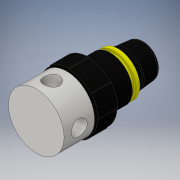
# Autodesk Inventor part: 101-3002-1
Saved by Autodesk Inventor 2016 SP2 (Build 200236200, 236)
## iProperties
Created: 2017-03-30
Part Number: 101-3002-1
Material: Aluminum
Document SubType Name: Modeling
Designer: smiku
Mass: 129.93 g
Surface Area: 139.496 cm^2
Volume: 48.1222 cm^3
Density: 2.7 g/cm^3
Appearance: Satin
Author: smiku
Autodesk Inventor part; units mm, degrees
ref_plane "YZ Plane" through (0, 0, 0) normal (1, 0, 0) x (0, 1, 0)
ref_plane "XY Plane" through (0, 0, 0) normal (0, 0, 1) x (1, 0, 0)
sketch "Sketch1" plane through (0, 0, 0) normal (0, 0, 1) x (1, 0, 0)
  circle A0 centre (0, 0) radius 17.9959
  dimension "d0" = 35.9918
  constraints: 1 centre point, 1 coincident
  measures "d0" diameter of A0
extrude "Extrusion1" add sketch "Sketch1" along normal blind 19.7358
sketch "Sketch2" plane through (0, 0, 0) normal (0, 0, -1) x (-1, 0, 0)
  circle A0 centre (0, 0) radius 12.7
  dimension "d3" = 25.4
  constraints: 1 centre point, 1 coincident
  measures "d3" diameter of A0
extrude "Extrusion2" add sketch "Sketch2" along normal blind 1.27
sketch "Sketch3" plane through (0, 0, -1.27) normal (0, 0, -1) x (-1, 0, 0)
  circle A0 centre (0, 0) radius 18.6055
  arc A1 (12.2451, 14.5931) -> (0, 19.05) centre (0, 0) ccw
  line L0 (0, 0) -> (12.2451, 14.5931) construction
  line L1 (0, 0) -> (0, 19.05) construction
  line L2 (0, 19.05) -> (0, 18.6055)
  line L3 (11.9594, 14.2526) -> (12.2451, 14.5931)
  arc A2 (11.9594, 14.2526) -> (0, 18.6055) centre (0, 0) ccw
  arc A3 (-14.5931, 12.2451) -> (-19.05, 0) centre (0, 0) ccw
  line L4 (-19.05, 0) -> (-18.6055, 0)
  arc A4 (-14.2526, 11.9594) -> (-18.6055, 0) centre (0, 0) ccw
  line L5 (-14.2526, 11.9594) -> (-14.5931, 12.2451)
  arc A5 (-12.2451, -14.5931) -> (0, -19.05) centre (0, 0) ccw
  line L6 (0, -19.05) -> (0, -18.6055)
  arc A6 (-11.9594, -14.2526) -> (0, -18.6055) centre (0, 0) ccw
  line L7 (-11.9594, -14.2526) -> (-12.2451, -14.5931)
  arc A7 (14.5931, -12.2451) -> (19.05, 0) centre (0, 0) ccw
  line L8 (19.05, 0) -> (18.6055, 0)
  arc A8 (14.2526, -11.9594) -> (18.6055, 0) centre (0, 0) ccw
  line L9 (14.2526, -11.9594) -> (14.5931, -12.2451)
  dimension "d6" = 37.211
  dimension "d7" = 19.05
  dimension "d8" = 40
  dimension "d11" = 360
  constraints: 20 end point, 18 point on circle, 9 centre point, 6 coincident, 2 point on line, 1 vertical, 41 other
  measures "d6" diameter of A0
  measures "d7" radius of A1
  measures "d8" angle of L0 L1
extrude "Extrusion3" add sketch "Sketch3" along normal blind 12.7 separate body
sketch "Sketch4" plane through (0, 0, -13.97) normal (0, 0, -1) x (-1, 0, 0)
  circle A0 centre (0, 0) radius 14.2875
  dimension "d15" = 28.575
  constraints: 1 centre point, 1 coincident
  measures "d15" diameter of A0
extrude "Extrusion4" add sketch "Sketch4" along normal blind 14.224 bodies 2
sketch "Sketch5" plane through (0, 0, -28.194) normal (0, 0, -1) x (-1, 0, 0)
  circle A0 centre (0, 0) radius 10.16
  dimension "d18" = 20.32
  constraints: 1 centre point, 1 coincident
  measures "d18" diameter of A0
extrude "Extrusion5" add sketch "Sketch5" along normal blind 10.16 bodies 2
sketch "Sketch6" plane through (0, 0, 0) normal (0, 1, 0) x (-1, 0, 0)
  line L0 (-10.16, -38.354) -> (10.16, -38.354) construction
  line L1 (0, -38.354) -> (11.7475, -38.354)
  line L2 (0, -38.354) -> (0, -49.784)
  line L3 (0, -49.784) -> (8.89, -49.784)
  arc A0 (8.89, -49.784) -> (10.795, -48.0569) centre (8.89, -47.8698) ccw
  line L4 (10.795, -48.0569) -> (11.7475, -38.354)
  point P0 (0, 0)
  dimension "d21" = 11.7475
  dimension "d22" = 11.43
  dimension "d23" = 8.89
  dimension "d24" = 10.795
  constraints: 8 end point, 2 horizontal, 2 point on circle, 2 tangent, 1 centre point, 1 midpoint, 1 vertical
  measures "d21" distance of L1.start L1.end
  measures "d22" distance of L1.start L2.end
  measures "d23" distance of L2.end L3.end
  measures "d24" distance from line of L2 L4.start
revolve "Revolution1" add sketch "Sketch6" angle 360 about axis through (0, 0, -38.354) along (0, 0, -1) bodies 2
sketch "Sketch7" plane through (0, 0, -28.194) normal (0, 0, -1) x (-1, 0, 0)
  circle A0 centre (0, 0) radius 10.16 projected
  circle A1 centre (0, 0) radius 12.7
  dimension "d26" = 25.4
  constraints: 1 centre point, 1 coincident
  measures "d26" diameter of A1
extrude "Extrusion6" add sketch "Sketch7" along normal blind 2.54 separate body
sketch "Sketch8" plane through (0, 0, -30.734) normal (0, 0, -1) x (-1, 0, 0)
  circle A0 centre (0, 0) radius 10.16 projected
  circle A1 centre (0, 0) radius 13.97
  dimension "d29" = 27.94
  constraints: 1 centre point, 1 coincident
  measures "d29" diameter of A1
extrude "Extrusion7" add sketch "Sketch8" along normal blind 2.54 bodies 3
ref_plane "Work Plane1" through (0, 17.9959, 0) normal (0, 1, 0) x (-1, 0, 0)
sketch "Sketch9" plane through (0, 17.9959, 0) normal (0, 1, 0) x (-1, 0, 0)
  line L0 (0, 0) -> (0, 19.7358) construction
  line L1 (17.9959, 19.7358) -> (-17.9959, 19.7358) construction
  circle A0 centre (0, 9.8679) radius 5.08
  dimension "d32" = 10.16
  constraints: 2 end point, 2 midpoint, 1 centre point
  measures "d32" diameter of A0
extrude "Extrusion8" cut sketch "Sketch9" against normal blind 15.24 bodies 1
pattern_circular "Circular Pattern1" count 4 over 360 about axis through (0, 0, 0) along (0, 0, 1) of "Extrusion8" bodies 1
body "Solid1"
body "Solid2"
body "Solid3"
